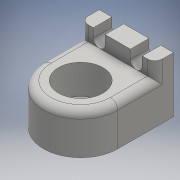
# Autodesk Inventor part: clip
Saved by Autodesk Inventor 2016 (Build 200138000, 138)
## iProperties
Created: 2016-02-21
Part Number: clip
Material: Generic
Document SubType Name: Modeling
Designer: Mikkel
Density: 1 g/cm^3
Appearance: Default
Author: Mikkel
Autodesk Inventor part; units mm, degrees
ref_plane "YZ Plane" through (0, 0, 0) normal (1, 0, 0) x (0, 1, 0)
ref_plane "XZ Plane" through (0, 0, 0) normal (0, 1, 0) x (-1, 0, 0)
ref_plane "XY Plane" through (0, 0, 0) normal (0, 0, 1) x (1, 0, 0)
sketch "Sketch1" plane through (0, 0, 0) normal (0, 0, 1) x (1, 0, 0)
  line L0 (20, 0) -> (20, 15)
  line L1 (20, 15) -> (0, 15)
  line L2 (0, 15) -> (0, 0)
  circle A0 centre (10, 0) radius 10
  circle A1 centre (10, 0) radius 2
  line L3 (0, 0) -> (8, 0)
  line L4 (12, 0) -> (20, 0)
  dimension "d3" = 20
  dimension "d4" = 15
  dimension "d5" = 4
  constraints: 10 end point, 3 parallel, 2 horizontal, 2 perpendicular, 2 point on circle, 1 centre point, 1 coincident, 1 horizontal alignment, 2 other
  measures "d3" distance of L1.end L0.end
  measures "d4" distance of L0.end L0.start
  measures "d5" diameter of A1
extrude "Extrusion1" add sketch "Sketch1" along normal blind 3 contours A0 L2 L1 L0 | L4 A1 L3 A0 | A0 L3 A1 L4
sketch "Sketch3" plane through (0, 0, 3) normal (0, 0, 1) x (1, 0, 0)
  circle A0 centre (10, 0) radius 2 projected
  circle A1 centre (10, 0) radius 6
  line L0 (0, 15) -> (0, 0) projected
  arc A2 (0, 0) -> (20, 0) centre (10, 0) ccw
  line L1 (0, 15) -> (20, 15)
  line L2 (20, 15) -> (20, 0)
  line L3 (0, 0) -> (0, 15)
  dimension "d8" = 12
  constraints: 6 end point, 3 point on circle, 2 centre point, 2 coincident, 1 horizontal, 1 parallel, 1 perpendicular
  measures "d8" diameter of A1
extrude "Extrusion2" add sketch "Sketch3" along normal blind 8 contours L1 L2 A2 L0
sketch "Sketch4" plane through (0, 0, 11) normal (0, 0, 1) x (1, 0, 0)
  line L0 (0, 15) -> (20, 15)
  line L1 (20, 15) -> (20, 10)
  line L2 (20, 10) -> (0, 10)
  line L3 (0, 10) -> (0, 15)
  line L4 (20, 15) -> (0, 15) projected
  point P0 (0, 0)
  dimension "d11" = 20
  dimension "d12" = 5
  constraints: 8 end point, 2 parallel, 1 collinear, 1 horizontal, 1 perpendicular
  measures "d11" distance of L1.end L2.end
  measures "d12" distance of L0.end L1.end
extrude "Extrusion3" add sketch "Sketch4" along normal blind 4
sketch "Sketch5" plane through (0, 10, 11) normal (0, -1, 0) x (1, 0, 0)
  circle A0 centre (5, 1.6) radius 1.6
  circle A1 centre (15, 1.6) radius 1.6
  line L0 (0, 0) -> (0, 4) projected
  line L1 (20, 0) -> (20, 4) projected
  line L2 (0, 4) -> (20, 4) projected
  line L3 (20, 0) -> (0, 0) projected
  line L4 (3.4, 1.6) -> (3.4, 4)
  line L5 (13.4, 1.6) -> (13.4, 4)
  line L6 (16.6, 1.6) -> (16.6, 4)
  line L7 (6.6, 1.6) -> (6.6, 4)
  point P0 (0, -11)
  dimension "d15" = 3.2
  dimension "d16" = 3.2
  dimension "d21" = 5
  dimension "d23" = 5
  constraints: 8 end point, 6 tangent, 4 point on circle, 4 point on line, 3 perpendicular, 2 centre point, 1 vertical
  measures "d15" diameter of A0
  measures "d16" diameter of A1
  measures "d21" distance from line of A0.centre L0
  measures "d23" distance from line of L1 A1.centre
extrude "Extrusion4" cut sketch "Sketch5" against normal through all contours A0 | A0 L4 L2 L7 | A1 | L2 L6 A1 L5
fillet "Fillet2" radius 2 5 edges at (0, 10, 13) (10, -10, 11) (20, 5, 11) (0, 5, 11) (20, 10, 13)
body "Solid1"
